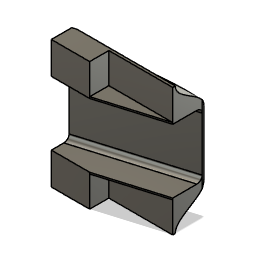
Abdeckung Motormount (Autodesk Fusion 360 design; units mm, degrees)
Autodesk Fusion 360 part; units mm, degrees
sketch "Skizze1" plane through (0, 0, 0) normal (0, 1, 0) x (1, 0, 0)
  line L0 (0, 0) -> (15, 0)
  line L1 (15, 0) -> (15, 8)
  line L2 (15, 8) -> (0, 8)
  line L3 (0, 8) -> (0, 0)
  line L4 (0, 8) -> (39.7107, 20)
  line L5 (39.7107, 20) -> (40, 19.0428)
  line L6 (40, 19.0428) -> (3.457, 8)
  line L7 (40, 19.0428) -> (40, 8)
  line L8 (40, 8) -> (15, 8)
  dimension "d1" = 15
  dimension "d2" = 8
  dimension "d3" = 1
  dimension "d4" = 20
  dimension "d5" = 40
  constraint horizontal L0
  constraint vertical L1
  constraint horizontal L2
  constraint vertical L3
  constraint coincident L0.start L3.end
  constraint perpendicular L4 L5
  constraint coincident L2 L6.end
  constraint parallel L4 L6
  constraint vertical L7
  constraint horizontal L8
  measures "d1" distance of L0.start L0.end
  measures "d2" distance of L0.start L2.end
  measures "d3" distance of L4 L6
  measures "d4" vertical distance of L0.end L4.end
  measures "d5" distance of L3 L5.end
extrude "Extrusion1" add sketch "Skizze1" along normal mid plane 50
ref_plane "Arbeitsebene1" through (39.8554, 0, -19.5214) normal (0.957249, 0, -0.289266) x (-0.289266, 0, -0.957249)
sketch "Skizze2" plane through (41.9259, 0, -12.6694) normal (0.957249, 0, -0.289266) x (-0.289266, 0, -0.957249)
  line L0 (6.658, 12.5) -> (-8.342, 12.5)
  line L1 (-8.342, 12.5) -> (-8.342, -12.5)
  line L2 (-8.342, -12.5) -> (6.658, -12.5)
  line L3 (6.658, -12.5) -> (6.658, 12.5)
  line L4 (6.658, 12.5) -> (-8.342, -12.5) construction
  line L5 (-8.342, 12.5) -> (6.658, -12.5) construction
  line L6 (6.658, -25) -> (6.658, 25)
  point P0 (-0.842, 0)
  dimension "d11" = 15
  dimension "d23" = 25
  constraint horizontal L0
  constraint perpendicular L0 L1
  constraint parallel L0 L2
  constraint parallel L1 L3
  constraint coincident L4 P0
  constraint coincident L5 P0
  constraint coincident L0.start L6
  constraint horizontal origin P0
  measures "d11" distance of L1.end L2.end
  measures "d23" distance of L0.end L1.end
extrude "Extrusion2" cut sketch "Skizze2" against normal blind 50
sketch "Skizze3" plane through (40, 0, 0) normal (1, 0, 0) x (0, 0, -1)
  line L0 (8, 12.5) -> (19.0428, 12.5)
  line L1 (19.0428, 12.5) -> (19.0428, 25)
  line L2 (19.0428, 25) -> (8, 25)
  line L3 (8, 25) -> (8, 12.5)
  line L4 (20, -25) -> (20, 25)
  line L5 (20, 25) -> (19.0428, 25)
  line L6 (19.0428, 25) -> (19.0428, 12.5)
  line L7 (19.0428, 12.5) -> (19.0428, -12.5)
  line L8 (19.0428, -12.5) -> (19.0428, -25)
  line L9 (19.0428, -25) -> (20, -25)
  line L10 (8, 12.5) -> (19.0428, 12.5)
  line L11 (19.0428, -12.5) -> (8, -12.5)
  line L12 (8, -12.5) -> (8, -25)
  line L13 (8, -25) -> (19.0428, -25)
  line L14 (19.0428, -25) -> (19.0428, -12.5)
  spline S0 degree 5 poles (20, -12.5) (20, -13.0888) (19.7652, -14.2211) (18.7091, -15.7836) (16.1706, -17.6488) (12.3294, -19.8512) (9.7909, -21.7164) (8.7348, -23.2789) (8.5, -24.4112) (8.5, -25) knots 0 0 0 0 0 0 0.2 0.4 0.6 0.8 1 1 1 1 1 1
  line L15 (20, -11.5) -> (20, -13.5)
  line L16 (8.5, -24) -> (8.5, -26)
  dimension "d14" = 2
  dimension "d15" = 2
  dimension "d16" = 0.5
  constraint coincident L4 S0.start
  constraint coincident L13 S0.end
  constraint midpoint S0.start L15
  constraint collinear L4 L15
  constraint horizontal L7.end S0.start
  constraint midpoint S0.end L16
  constraint parallel L4 L16
  measures "d14" distance of L15.start L15.end
  measures "d15" distance of L16.start L16.end
  measures "d16" distance of L12 L16
extrude "Extrusion3" cut sketch "Skizze3" against normal blind 50 contours L4 L8 L9 L14 S0 L15 | L8 L13 L14 S0
extrude "Extrusion4" add 2 faces at (31.6667, -16.6667, -8) (31.6667, 16.6667, -8) along direction (0, 0, 1) blind 0.5
mirror "Spiegeln1" about plane through (0, 0, 0) normal (0, 1, 0) of "Extrusion3"
fillet "Abrundung1" radius 2 2 edges at (20, -12.5, -12.999) (20, 12.5, -12.999)
sketch "Skizze4" plane through (0, 12.5, 0) normal (0, -1, 0) x (1, 0, 0)
  line L0 (0, -4.866) -> (40, -16.9534)
  line L1 (40, -16.9534) -> (40, -7.5)
  line L2 (40, -7.5) -> (15, -7.5)
  line L3 (15, -7.5) -> (15, 0)
  line L4 (15, 0) -> (0, 0)
  line L5 (0, 0) -> (0, -4.866)
  line L6 (15, 0) -> (40, -7.5)
  constraint coincident L3.end L4.start
  constraint coincident L1.end L2.start
extrude "Extrusion5" add sketch "Skizze4" against normal blind 0.6 contours L2 L3 L6
mirror "Spiegeln2" about plane through (0, 0, 0) normal (0, 1, 0) of "Extrusion5"
equation "d15 = d14"
